Autodesk Fusion 360 part; units mm, degrees
(part 2 of 3)
  spline S192 degree 2 poles (79.2808, -26.577) (79.6552, -26.1242) (80.3974, -26.1242) knots 0 0 0 1 1 1
  spline S193 degree 2 poles (81.8524, -24.5056) (82.3952, -24.5056) (82.6732, -24.3274) knots 0 0 0 1 1 1
  spline S194 degree 2 poles (82.6732, -24.3274) (82.9511, -24.1492) (82.9511, -23.7471) knots 0 0 0 1 1 1
  spline S195 degree 2 poles (82.9511, -23.7471) (82.9511, -23.3481) (82.6748, -23.1732) knots 0 0 0 1 1 1
  spline S196 degree 2 poles (82.6748, -23.1732) (82.3985, -22.9983) (81.8524, -22.9983) knots 0 0 0 1 1 1
  spline S197 degree 2 poles (81.8524, -22.9983) (81.3097, -22.9983) (81.0383, -23.1748) knots 0 0 0 1 1 1
  spline S198 degree 2 poles (81.0383, -23.1748) (80.7669, -23.3514) (80.7669, -23.7536) knots 0 0 0 1 1 1
  spline S199 degree 2 poles (80.7669, -23.7536) (80.7669, -24.1525) (81.0366, -24.3291) knots 0 0 0 1 1 1
  spline S200 degree 2 poles (81.0366, -24.3291) (81.3064, -24.5056) (81.8524, -24.5056) knots 0 0 0 1 1 1
  spline S201 degree 2 poles (81.8524, -21.9781) (82.7451, -21.9781) (83.2486, -22.449) knots 0 0 0 1 1 1
  spline S202 degree 2 poles (83.2486, -22.449) (83.7522, -22.9198) (83.7522, -23.7601) knots 0 0 0 1 1 1
  spline S203 degree 2 poles (83.7522, -23.7601) (83.7522, -24.2866) (83.5217, -24.6887) knots 0 0 0 1 1 1
  spline S204 degree 2 poles (83.5217, -24.6887) (83.2911, -25.0909) (82.8595, -25.3067) knots 0 0 0 1 1 1
  spline S205 degree 2 poles (82.8595, -25.3067) (82.4279, -25.5225) (81.8524, -25.5225) knots 0 0 0 1 1 1
  spline S206 degree 2 poles (81.8524, -25.5225) (80.9565, -25.5225) (80.4595, -25.055) knots 0 0 0 1 1 1
  spline S207 degree 2 poles (80.4595, -25.055) (79.9625, -24.5874) (79.9625, -23.7405) knots 0 0 0 1 1 1
  spline S208 degree 2 poles (79.9625, -23.7405) (79.9625, -23.2141) (80.1914, -22.8119) knots 0 0 0 1 1 1
  spline S209 degree 2 poles (80.1914, -22.8119) (80.4203, -22.4097) (80.8486, -22.1939) knots 0 0 0 1 1 1
  spline S210 degree 2 poles (80.8486, -22.1939) (81.277, -21.9781) (81.8524, -21.9781) knots 0 0 0 1 1 1
  line L170 (83.6868, -18.1492) -> (82.4083, -18.4304)
  line L171 (82.4083, -18.4304) -> (80.793, -18.8097)
  line L172 (80.793, -18.8097) -> (80.793, -18.8326)
  line L173 (80.793, -18.8326) -> (83.6868, -19.4996)
  line L174 (83.6868, -19.4996) -> (83.6868, -20.5721)
  line L175 (83.6868, -20.5721) -> (80.0312, -21.6119)
  line L176 (80.0312, -21.6119) -> (80.0312, -20.6179)
  line L177 (80.0312, -20.6179) -> (81.6497, -20.1961)
  spline S211 degree 2 poles (81.6497, -20.1961) (82.0846, -20.0947) (82.8497, -19.9901) knots 0 0 0 1 1 1
  line L178 (82.8497, -19.9901) -> (82.8497, -19.9705)
  spline S212 degree 2 poles (82.8497, -19.9705) (82.6012, -19.9574) (82.0617, -19.856) knots 0 0 0 1 1 1
  line L179 (82.0617, -19.856) -> (81.7838, -19.8037)
  line L180 (81.7838, -19.8037) -> (80.0312, -19.3525)
  line L181 (80.0312, -19.3525) -> (80.0312, -18.2539)
  line L182 (80.0312, -18.2539) -> (81.7838, -17.8255)
  spline S213 degree 2 poles (81.7838, -17.8255) (81.8557, -17.8124) (81.9963, -17.7847) knots 0 0 0 1 1 1
  spline S214 degree 2 poles (81.9963, -17.7847) (82.1369, -17.7569) (82.2955, -17.7307) knots 0 0 0 1 1 1
  spline S215 degree 2 poles (82.2955, -17.7307) (82.4541, -17.7045) (82.6061, -17.6833) knots 0 0 0 1 1 1
  spline S216 degree 2 poles (82.6061, -17.6833) (82.7582, -17.662) (82.8497, -17.6588) knots 0 0 0 1 1 1
  line L183 (82.8497, -17.6588) -> (82.8497, -17.6392)
  spline S217 degree 2 poles (82.8497, -17.6392) (82.6143, -17.6097) (82.2039, -17.5345) knots 0 0 0 1 1 1
  spline S218 degree 2 poles (82.2039, -17.5345) (81.7936, -17.4593) (81.6497, -17.4266) knots 0 0 0 1 1 1
  line L184 (81.6497, -17.4266) -> (80.0312, -16.9885)
  line L185 (80.0312, -16.9885) -> (80.0312, -16.0108)
  line L186 (80.0312, -16.0108) -> (83.6868, -17.0637)
  line L187 (83.6868, -17.0637) -> (83.6868, -18.1492)
  spline S219 degree 2 poles (80.6721, -13.9084) (80.6721, -14.2255) (80.8732, -14.4054) knots 0 0 0 1 1 1
  spline S220 degree 2 poles (80.8732, -14.4054) (81.0742, -14.5852) (81.4437, -14.6114) knots 0 0 0 1 1 1
  line L188 (81.4437, -14.6114) -> (81.4437, -13.2119)
  spline S221 degree 2 poles (81.4437, -13.2119) (81.0742, -13.2184) (80.8732, -13.4048) knots 0 0 0 1 1 1
  spline S222 degree 2 poles (80.8732, -13.4048) (80.6721, -13.5912) (80.6721, -13.9084) knots 0 0 0 1 1 1
  spline S223 degree 2 poles (83.7522, -13.7678) (83.7522, -14.6506) (83.265, -15.1476) knots 0 0 0 1 1 1
  spline S224 degree 2 poles (83.265, -15.1476) (82.7778, -15.6446) (81.8851, -15.6446) knots 0 0 0 1 1 1
  spline S225 degree 2 poles (81.8851, -15.6446) (80.9663, -15.6446) (80.4644, -15.1852) knots 0 0 0 1 1 1
  spline S226 degree 2 poles (80.4644, -15.1852) (79.9625, -14.7258) (79.9625, -13.9149) knots 0 0 0 1 1 1
  spline S227 degree 2 poles (79.9625, -13.9149) (79.9625, -13.14) (80.4039, -12.7084) knots 0 0 0 1 1 1
  spline S228 degree 2 poles (80.4039, -12.7084) (80.8454, -12.2768) (81.6236, -12.2768) knots 0 0 0 1 1 1
  line L189 (81.6236, -12.2768) -> (82.1075, -12.2768)
  line L190 (82.1075, -12.2768) -> (82.1075, -14.6342)
  spline S229 degree 2 poles (82.1075, -14.6342) (82.5326, -14.6179) (82.7712, -14.3825) knots 0 0 0 1 1 1
  spline S230 degree 2 poles (82.7712, -14.3825) (83.0099, -14.1471) (83.0099, -13.722) knots 0 0 0 1 1 1
  spline S231 degree 2 poles (83.0099, -13.722) (83.0099, -13.3917) (82.9413, -13.0975) knots 0 0 0 1 1 1
  spline S232 degree 2 poles (82.9413, -13.0975) (82.8726, -12.8032) (82.7222, -12.4827) knots 0 0 0 1 1 1
  line L191 (82.7222, -12.4827) -> (83.4939, -12.4827)
  spline S233 degree 2 poles (83.4939, -12.4827) (83.6246, -12.7443) (83.6884, -13.0419) knots 0 0 0 1 1 1
  spline S234 degree 2 poles (83.6884, -13.0419) (83.7522, -13.3394) (83.7522, -13.7678) knots 0 0 0 1 1 1
  spline S235 degree 2 poles (79.9625, -9.4255) (79.9625, -9.2228) (79.992, -9.0887) knots 0 0 0 1 1 1
  line L192 (79.992, -9.0887) -> (80.9271, -9.1639)
  spline S236 degree 2 poles (80.9271, -9.1639) (80.8944, -9.2849) (80.8944, -9.4582) knots 0 0 0 1 1 1
  spline S237 degree 2 poles (80.8944, -9.4582) (80.8944, -9.9356) (81.1396, -10.2021) knots 0 0 0 1 1 1
  spline S238 degree 2 poles (81.1396, -10.2021) (81.3849, -10.4686) (81.8263, -10.4686) knots 0 0 0 1 1 1
  line L193 (81.8263, -10.4686) -> (83.6868, -10.4686)
  line L194 (83.6868, -10.4686) -> (83.6868, -11.4659)
  line L195 (83.6868, -11.4659) -> (80.0312, -11.4659)
  line L196 (80.0312, -11.4659) -> (80.0312, -10.7105)
  line L197 (80.0312, -10.7105) -> (80.6459, -10.5634)
  line L198 (80.6459, -10.5634) -> (80.6459, -10.5144)
  spline S239 degree 2 poles (80.6459, -10.5144) (80.3385, -10.3443) (80.1505, -10.055) knots 0 0 0 1 1 1
  spline S240 degree 2 poles (80.1505, -10.055) (79.9625, -9.7656) (79.9625, -9.4255) knots 0 0 0 1 1 1
  line L199 (86.415, -25.4932) -> (89.5081, -25.4932)
  spline S241 degree 2 poles (89.5081, -25.4932) (90.0378, -25.4932) (90.4368, -25.7303) knots 0 0 0 1 1 1
  spline S242 degree 2 poles (90.4368, -25.7303) (90.8357, -25.9673) (91.0482, -26.4153) knots 0 0 0 1 1 1
  spline S243 degree 2 poles (91.0482, -26.4153) (91.2607, -26.8632) (91.2607, -27.4747) knots 0 0 0 1 1 1
  spline S244 degree 2 poles (91.2607, -27.4747) (91.2607, -28.3968) (90.7883, -28.9068) knots 0 0 0 1 1 1
  spline S245 degree 2 poles (90.7883, -28.9068) (90.3158, -29.4169) (89.4951, -29.4169) knots 0 0 0 1 1 1
  line L200 (89.4951, -29.4169) -> (86.415, -29.4169)
  line L201 (86.415, -29.4169) -> (86.415, -28.4066)
  line L202 (86.415, -28.4066) -> (89.3414, -28.4066)
  spline S246 degree 2 poles (89.3414, -28.4066) (89.894, -28.4066) (90.1523, -28.1842) knots 0 0 0 1 1 1
  spline S247 degree 2 poles (90.1523, -28.1842) (90.4106, -27.9619) (90.4106, -27.4485) knots 0 0 0 1 1 1
  spline S248 degree 2 poles (90.4106, -27.4485) (90.4106, -26.9515) (90.1506, -26.7276) knots 0 0 0 1 1 1
  spline S249 degree 2 poles (90.1506, -26.7276) (89.8907, -26.5036) (89.3348, -26.5036) knots 0 0 0 1 1 1
  line L203 (89.3348, -26.5036) -> (86.415, -26.5036)
  line L204 (86.415, -26.5036) -> (86.415, -25.4932)
  spline S250 degree 2 poles (89.8678, -21.5009) (90.5152, -21.5009) (90.888, -21.9668) knots 0 0 0 1 1 1
  spline S251 degree 2 poles (90.888, -21.9668) (91.2607, -22.4327) (91.2607, -23.2632) knots 0 0 0 1 1 1
  spline S252 degree 2 poles (91.2607, -23.2632) (91.2607, -24.0284) (90.973, -24.6169) knots 0 0 0 1 1 1
  line L205 (90.973, -24.6169) -> (90.0313, -24.6169)
  spline S253 degree 2 poles (90.0313, -24.6169) (90.2471, -24.133) (90.3354, -23.7979) knots 0 0 0 1 1 1
  spline S254 degree 2 poles (90.3354, -23.7979) (90.4237, -23.4627) (90.4237, -23.1848) knots 0 0 0 1 1 1
  spline S255 degree 2 poles (90.4237, -23.1848) (90.4237, -22.8513) (90.2962, -22.6731) knots 0 0 0 1 1 1
  spline S256 degree 2 poles (90.2962, -22.6731) (90.1686, -22.4949) (89.9169, -22.4949) knots 0 0 0 1 1 1
  spline S257 degree 2 poles (89.9169, -22.4949) (89.7763, -22.4949) (89.6667, -22.5733) knots 0 0 0 1 1 1
  spline S258 degree 2 poles (89.6667, -22.5733) (89.5572, -22.6518) (89.4558, -22.8038) knots 0 0 0 1 1 1
  spline S259 degree 2 poles (89.4558, -22.8038) (89.3545, -22.9559) (89.1321, -23.4235) knots 0 0 0 1 1 1
  spline S260 degree 2 poles (89.1321, -23.4235) (88.9261, -23.8616) (88.7365, -24.0807) knots 0 0 0 1 1 1
  spline S261 degree 2 poles (88.7365, -24.0807) (88.5468, -24.2998) (88.2951, -24.4306) knots 0 0 0 1 1 1
  spline S262 degree 2 poles (88.2951, -24.4306) (88.0433, -24.5613) (87.7065, -24.5613) knots 0 0 0 1 1 1
  spline S263 degree 2 poles (87.7065, -24.5613) (87.0722, -24.5613) (86.7092, -24.1314) knots 0 0 0 1 1 1
  spline S264 degree 2 poles (86.7092, -24.1314) (86.3463, -23.7014) (86.3463, -22.9428) knots 0 0 0 1 1 1
  spline S265 degree 2 poles (86.3463, -22.9428) (86.3463, -22.5701) (86.4346, -22.2316) knots 0 0 0 1 1 1
  spline S266 degree 2 poles (86.4346, -22.2316) (86.5229, -21.8932) (86.6831, -21.5237) knots 0 0 0 1 1 1
  line L206 (86.6831, -21.5237) -> (87.4711, -21.8507)
  spline S267 degree 2 poles (87.4711, -21.8507) (87.3141, -22.2333) (87.252, -22.4834) knots 0 0 0 1 1 1
  spline S268 degree 2 poles (87.252, -22.4834) (87.1899, -22.7335) (87.1899, -22.9755) knots 0 0 0 1 1 1
  spline S269 degree 2 poles (87.1899, -22.9755) (87.1899, -23.2632) (87.3239, -23.4169) knots 0 0 0 1 1 1
  spline S270 degree 2 poles (87.3239, -23.4169) (87.458, -23.5706) (87.6738, -23.5706) knots 0 0 0 1 1 1
  spline S271 degree 2 poles (87.6738, -23.5706) (87.8079, -23.5706) (87.9076, -23.5085) knots 0 0 0 1 1 1
  spline S272 degree 2 poles (87.9076, -23.5085) (88.0073, -23.4464) (88.1005, -23.3107) knots 0 0 0 1 1 1
  spline S273 degree 2 poles (88.1005, -23.3107) (88.1937, -23.175) (88.4357, -22.6682) knots 0 0 0 1 1 1
  spline S274 degree 2 poles (88.4357, -22.6682) (88.7561, -21.9979) (89.0782, -21.7494) knots 0 0 0 1 1 1
  spline S275 degree 2 poles (89.0782, -21.7494) (89.4002, -21.5009) (89.8678, -21.5009) knots 0 0 0 1 1 1
  line L207 (86.415, -20.6344) -> (86.415, -19.1466)
  spline S276 degree 2 poles (86.415, -19.1466) (86.415, -18.1297) (86.7043, -17.6703) knots 0 0 0 1 1 1
  spline S277 degree 2 poles (86.7043, -17.6703) (86.9937, -17.2109) (87.6248, -17.2109) knots 0 0 0 1 1 1
  spline S278 degree 2 poles (87.6248, -17.2109) (88.0531, -17.2109) (88.3278, -17.412) knots 0 0 0 1 1 1
  spline S279 degree 2 poles (88.3278, -17.412) (88.6024, -17.6131) (88.658, -17.9466) knots 0 0 0 1 1 1
  line L208 (88.658, -17.9466) -> (88.6907, -17.9466)
  spline S280 degree 2 poles (88.6907, -17.9466) (88.7921, -17.4921) (89.07, -17.291) knots 0 0 0 1 1 1
  spline S281 degree 2 poles (89.07, -17.291) (89.3479, -17.09) (89.809, -17.09) knots 0 0 0 1 1 1
  spline S282 degree 2 poles (89.809, -17.09) (90.4629, -17.09) (90.8291, -17.5624) knots 0 0 0 1 1 1
  spline S283 degree 2 poles (90.8291, -17.5624) (91.1953, -18.0349) (91.1953, -18.8458) knots 0 0 0 1 1 1
  line L209 (91.1953, -18.8458) -> (91.1953, -20.6344)
  line L210 (91.1953, -20.6344) -> (86.415, -20.6344)
  line L211 (88.3081, -19.6207) -> (88.3081, -19.0322)
  spline S284 degree 2 poles (88.3081, -19.0322) (88.3081, -18.6202) (88.1806, -18.4355) knots 0 0 0 1 1 1
  spline S285 degree 2 poles (88.1806, -18.4355) (88.0531, -18.2507) (87.7588, -18.2507) knots 0 0 0 1 1 1
  spline S286 degree 2 poles (87.7588, -18.2507) (87.4842, -18.2507) (87.3648, -18.4518) knots 0 0 0 1 1 1
  spline S287 degree 2 poles (87.3648, -18.4518) (87.2455, -18.6529) (87.2455, -19.0878) knots 0 0 0 1 1 1
  line L212 (87.2455, -19.0878) -> (87.2455, -19.6207)
  line L213 (87.2455, -19.6207) -> (88.3081, -19.6207)
  line L214 (89.1125, -19.6207) -> (90.3583, -19.6207)
  line L215 (90.3583, -19.6207) -> (90.3583, -18.9603)
  spline S288 degree 2 poles (90.3583, -18.9603) (90.3583, -18.5417) (90.1981, -18.3423) knots 0 0 0 1 1 1
  spline S289 degree 2 poles (90.1981, -18.3423) (90.0378, -18.1428) (89.7076, -18.1428) knots 0 0 0 1 1 1
  spline S290 degree 2 poles (89.7076, -18.1428) (89.1125, -18.1428) (89.1125, -18.9929) knots 0 0 0 1 1 1
  line L216 (89.1125, -18.9929) -> (89.1125, -19.6207)
  spline S291 degree 2 poles (88.775, -9.3627) (89.9554, -9.3627) (90.5832, -10.0346) knots 0 0 0 1 1 1
  spline S292 degree 2 poles (90.5832, -10.0346) (91.211, -10.7066) (91.211, -11.9752) knots 0 0 0 1 1 1
  line L217 (91.211, -11.9752) -> (91.211, -13.3289)
  line L218 (91.211, -13.3289) -> (86.4306, -13.3289)
  line L219 (86.4306, -13.3289) -> (86.4306, -11.8281)
  spline S293 degree 2 poles (86.4306, -11.8281) (86.4306, -10.6575) (87.0486, -10.0101) knots 0 0 0 1 1 1
  spline S294 degree 2 poles (87.0486, -10.0101) (87.6666, -9.3627) (88.775, -9.3627) knots 0 0 0 1 1 1
  spline S295 degree 2 poles (88.8012, -10.4156) (87.2611, -10.4156) (87.2611, -11.7758) knots 0 0 0 1 1 1
  line L220 (87.2611, -11.7758) -> (87.2611, -12.3153)
  line L221 (87.2611, -12.3153) -> (90.3739, -12.3153)
  line L222 (90.3739, -12.3153) -> (90.3739, -11.8804)
  spline S296 degree 2 poles (90.3739, -11.8804) (90.3739, -10.4156) (88.8012, -10.4156) knots 0 0 0 1 1 1
  spline S297 degree 2 poles (87.2055, -6.3415) (87.2055, -6.9137) (87.6355, -7.2276) knots 0 0 0 1 1 1
  spline S298 degree 2 poles (87.6355, -7.2276) (88.0655, -7.5415) (88.8339, -7.5415) knots 0 0 0 1 1 1
  spline S299 degree 2 poles (88.8339, -7.5415) (90.4328, -7.5415) (90.4328, -6.3415) knots 0 0 0 1 1 1
  spline S300 degree 2 poles (90.4328, -6.3415) (90.4328, -5.8379) (90.181, -5.1218) knots 0 0 0 1 1 1
  line L223 (90.181, -5.1218) -> (91.0312, -5.1218)
  spline S301 degree 2 poles (91.0312, -5.1218) (91.2764, -5.7104) (91.2764, -6.4363) knots 0 0 0 1 1 1
  spline S302 degree 2 poles (91.2764, -6.4363) (91.2764, -7.4793) (90.6437, -8.0319) knots 0 0 0 1 1 1
  spline S303 degree 2 poles (90.6437, -8.0319) (90.011, -8.5845) (88.8273, -8.5845) knots 0 0 0 1 1 1
  spline S304 degree 2 poles (88.8273, -8.5845) (88.0818, -8.5845) (87.5211, -8.3131) knots 0 0 0 1 1 1
  spline S305 degree 2 poles (87.5211, -8.3131) (86.9603, -8.0417) (86.6611, -7.5333) knots 0 0 0 1 1 1
  spline S306 degree 2 poles (86.6611, -7.5333) (86.3619, -7.0248) (86.3619, -6.3415) knots 0 0 0 1 1 1
  spline S307 degree 2 poles (86.3619, -6.3415) (86.3619, -5.645) (86.6987, -4.942) knots 0 0 0 1 1 1
  line L224 (86.6987, -4.942) -> (87.5227, -5.269)
  spline S308 degree 2 poles (87.5227, -5.269) (87.3952, -5.5371) (87.3004, -5.8085) knots 0 0 0 1 1 1
  spline S309 degree 2 poles (87.3004, -5.8085) (87.2055, -6.0799) (87.2055, -6.3415) knots 0 0 0 1 1 1
  line L225 (91.0279, -57.901) -> (91.0279, -58.9146)
  line L226 (91.0279, -58.9146) -> (87.0912, -58.9146)
  line L227 (87.0912, -58.9146) -> (87.0912, -60.2127)
  line L228 (87.0912, -60.2127) -> (86.2476, -60.2127)
  line L229 (86.2476, -60.2127) -> (86.2476, -56.6029)
  line L230 (86.2476, -56.6029) -> (87.0912, -56.6029)
  line L231 (87.0912, -56.6029) -> (87.0912, -57.901)
  line L232 (87.0912, -57.901) -> (91.0279, -57.901)
  line L233 (91.0279, -54.0231) -> (91.0279, -55.0367)
  line L234 (91.0279, -55.0367) -> (87.0912, -55.0367)
  line L235 (87.0912, -55.0367) -> (87.0912, -56.3348)
  line L236 (87.0912, -56.3348) -> (86.2476, -56.3348)
  line L237 (86.2476, -56.3348) -> (86.2476, -52.725)
  line L238 (86.2476, -52.725) -> (87.0912, -52.725)
  line L239 (87.0912, -52.725) -> (87.0912, -54.0231)
  line L240 (87.0912, -54.0231) -> (91.0279, -54.0231)
  line L241 (91.0279, -51.9893) -> (86.2476, -51.9893)
  line L242 (86.2476, -51.9893) -> (86.2476, -50.9757)
  line L243 (86.2476, -50.9757) -> (90.1909, -50.9757)
  line L244 (90.1909, -50.9757) -> (90.1909, -49.0367)
  line L245 (90.1909, -49.0367) -> (91.0279, -49.0367)
  line L246 (91.0279, -49.0367) -> (91.0279, -51.9893)
  line L247 (88.4448, -91.7143) -> (88.4448, -91.3873)
  spline S310 degree 2 poles (88.4448, -91.3873) (88.4448, -90.9067) (88.2846, -90.6778) knots 0 0 0 1 1 1
  spline S311 degree 2 poles (88.2846, -90.6778) (88.1244, -90.4489) (87.781, -90.4489) knots 0 0 0 1 1 1
  spline S312 degree 2 poles (87.781, -90.4489) (87.441, -90.4489) (87.2971, -90.6827) knots 0 0 0 1 1 1
  spline S313 degree 2 poles (87.2971, -90.6827) (87.1532, -90.9165) (87.1532, -91.4069) knots 0 0 0 1 1 1
  line L248 (87.1532, -91.4069) -> (87.1532, -91.7143)
  line L249 (87.1532, -91.7143) -> (88.4448, -91.7143)
  line L250 (89.2688, -91.7143) -> (91.1031, -91.7143)
  line L251 (91.1031, -91.7143) -> (91.1031, -92.7279)
  line L252 (91.1031, -92.7279) -> (86.3227, -92.7279)
  line L253 (86.3227, -92.7279) -> (86.3227, -91.335)
  spline S314 degree 2 poles (86.3227, -91.335) (86.3227, -90.3606) (86.6775, -89.893) knots 0 0 0 1 1 1
  spline S315 degree 2 poles (86.6775, -89.893) (87.0323, -89.4255) (87.7549, -89.4255) knots 0 0 0 1 1 1
  spline S316 degree 2 poles (87.7549, -89.4255) (88.1767, -89.4255) (88.5053, -89.6576) knots 0 0 0 1 1 1
  spline S317 degree 2 poles (88.5053, -89.6576) (88.8339, -89.8898) (89.0203, -90.3148) knots 0 0 0 1 1 1
  spline S318 degree 2 poles (89.0203, -90.3148) (90.6323, -89.2358) (91.1031, -88.9088) knots 0 0 0 1 1 1
  line L254 (91.1031, -88.9088) -> (91.1031, -90.0336)
  line L255 (91.1031, -90.0336) -> (89.2688, -91.1748)
  line L256 (89.2688, -91.1748) -> (89.2688, -91.7143)
  spline S319 degree 2 poles (89.7756, -85.4854) (90.423, -85.4854) (90.7957, -85.9514) knots 0 0 0 1 1 1
  spline S320 degree 2 poles (90.7957, -85.9514) (91.1685, -86.4173) (91.1685, -87.2478) knots 0 0 0 1 1 1
  spline S321 degree 2 poles (91.1685, -87.2478) (91.1685, -88.0129) (90.8808, -88.6015) knots 0 0 0 1 1 1
  line L257 (90.8808, -88.6015) -> (89.9391, -88.6015)
  spline S322 degree 2 poles (89.9391, -88.6015) (90.1549, -88.1176) (90.2432, -87.7824) knots 0 0 0 1 1 1
  spline S323 degree 2 poles (90.2432, -87.7824) (90.3314, -87.4473) (90.3314, -87.1693) knots 0 0 0 1 1 1
  spline S324 degree 2 poles (90.3314, -87.1693) (90.3314, -86.8358) (90.2039, -86.6576) knots 0 0 0 1 1 1
  spline S325 degree 2 poles (90.2039, -86.6576) (90.0764, -86.4794) (89.8246, -86.4794) knots 0 0 0 1 1 1
  spline S326 degree 2 poles (89.8246, -86.4794) (89.684, -86.4794) (89.5745, -86.5579) knots 0 0 0 1 1 1
  spline S327 degree 2 poles (89.5745, -86.5579) (89.465, -86.6364) (89.3636, -86.7884) knots 0 0 0 1 1 1
  spline S328 degree 2 poles (89.3636, -86.7884) (89.2622, -86.9405) (89.0399, -87.408) knots 0 0 0 1 1 1
  spline S329 degree 2 poles (89.0399, -87.408) (88.8339, -87.8462) (88.6442, -88.0652) knots 0 0 0 1 1 1
  spline S330 degree 2 poles (88.6442, -88.0652) (88.4546, -88.2843) (88.2028, -88.4151) knots 0 0 0 1 1 1
  spline S331 degree 2 poles (88.2028, -88.4151) (87.9511, -88.5459) (87.6143, -88.5459) knots 0 0 0 1 1 1
  spline S332 degree 2 poles (87.6143, -88.5459) (86.9799, -88.5459) (86.617, -88.1159) knots 0 0 0 1 1 1
  spline S333 degree 2 poles (86.617, -88.1159) (86.2541, -87.686) (86.2541, -86.9274) knots 0 0 0 1 1 1
  spline S334 degree 2 poles (86.2541, -86.9274) (86.2541, -86.5546) (86.3423, -86.2162) knots 0 0 0 1 1 1
  spline S335 degree 2 poles (86.3423, -86.2162) (86.4306, -85.8778) (86.5908, -85.5083) knots 0 0 0 1 1 1
  line L258 (86.5908, -85.5083) -> (87.3788, -85.8353)
  spline S336 degree 2 poles (87.3788, -85.8353) (87.2219, -86.2178) (87.1598, -86.468) knots 0 0 0 1 1 1
  spline S337 degree 2 poles (87.1598, -86.468) (87.0976, -86.7181) (87.0976, -86.9601) knots 0 0 0 1 1 1
  spline S338 degree 2 poles (87.0976, -86.9601) (87.0976, -87.2478) (87.2317, -87.4015) knots 0 0 0 1 1 1
  spline S339 degree 2 poles (87.2317, -87.4015) (87.3658, -87.5552) (87.5816, -87.5552) knots 0 0 0 1 1 1
  spline S340 degree 2 poles (87.5816, -87.5552) (87.7156, -87.5552) (87.8154, -87.493) knots 0 0 0 1 1 1
  spline S341 degree 2 poles (87.8154, -87.493) (87.9151, -87.4309) (88.0083, -87.2952) knots 0 0 0 1 1 1
  spline S342 degree 2 poles (88.0083, -87.2952) (88.1015, -87.1595) (88.3434, -86.6527) knots 0 0 0 1 1 1
  spline S343 degree 2 poles (88.3434, -86.6527) (88.6639, -85.9824) (88.9859, -85.7339) knots 0 0 0 1 1 1
  spline S344 degree 2 poles (88.9859, -85.7339) (89.308, -85.4854) (89.7756, -85.4854) knots 0 0 0 1 1 1
  line L259 (91.1031, -81.6108) -> (91.1031, -84.9524)
  line L260 (91.1031, -84.9524) -> (90.4001, -84.9524)
  line L261 (90.4001, -84.9524) -> (89.187, -83.7524)
  spline S345 degree 2 poles (89.187, -83.7524) (88.641, -83.2195) (88.4301, -83.056) knots 0 0 0 1 1 1
  spline S346 degree 2 poles (88.4301, -83.056) (88.2192, -82.8925) (88.0393, -82.8206) knots 0 0 0 1 1 1
  spline S347 degree 2 poles (88.0393, -82.8206) (87.8595, -82.7486) (87.6666, -82.7486) knots 0 0 0 1 1 1
  spline S348 degree 2 poles (87.6666, -82.7486) (87.3788, -82.7486) (87.2382, -82.9072) knots 0 0 0 1 1 1
  spline S349 degree 2 poles (87.2382, -82.9072) (87.0976, -83.0658) (87.0976, -83.3306) knots 0 0 0 1 1 1
  spline S350 degree 2 poles (87.0976, -83.3306) (87.0976, -83.6086) (87.2252, -83.8702) knots 0 0 0 1 1 1
  spline S351 degree 2 poles (87.2252, -83.8702) (87.3527, -84.1317) (87.5881, -84.4162) knots 0 0 0 1 1 1
  line L262 (87.5881, -84.4162) -> (86.9374, -84.9655)
  spline S352 degree 2 poles (86.9374, -84.9655) (86.6366, -84.6124) (86.5124, -84.3802) knots 0 0 0 1 1 1
  spline S353 degree 2 poles (86.5124, -84.3802) (86.3881, -84.1481) (86.3211, -83.8734) knots 0 0 0 1 1 1
  spline S354 degree 2 poles (86.3211, -83.8734) (86.2541, -83.5988) (86.2541, -83.2587) knots 0 0 0 1 1 1
  spline S355 degree 2 poles (86.2541, -83.2587) (86.2541, -82.8108) (86.4175, -82.4674) knots 0 0 0 1 1 1
  spline S356 degree 2 poles (86.4175, -82.4674) (86.581, -82.1241) (86.8753, -81.9345) knots 0 0 0 1 1 1
  spline S357 degree 2 poles (86.8753, -81.9345) (87.1696, -81.7448) (87.5489, -81.7448) knots 0 0 0 1 1 1
  spline S358 degree 2 poles (87.5489, -81.7448) (87.8791, -81.7448) (88.1685, -81.8609) knots 0 0 0 1 1 1
  spline S359 degree 2 poles (88.1685, -81.8609) (88.4579, -81.977) (88.762, -82.2206) knots 0 0 0 1 1 1
  spline S360 degree 2 poles (88.762, -82.2206) (89.066, -82.4642) (89.6284, -83.0789) knots 0 0 0 1 1 1
  line L263 (89.6284, -83.0789) -> (90.2072, -83.6936)
  line L264 (90.2072, -83.6936) -> (90.253, -83.6936)
  line L265 (90.253, -83.6936) -> (90.253, -81.6108)
  line L266 (90.253, -81.6108) -> (91.1031, -81.6108)
  spline S361 degree 2 poles (87.3919, -77.9748) (87.8399, -77.9748) (88.1538, -78.2462) knots 0 0 0 1 1 1
  spline S362 degree 2 poles (88.1538, -78.2462) (88.4677, -78.5176) (88.5854, -79.008) knots 0 0 0 1 1 1
  line L267 (88.5854, -79.008) -> (88.605, -79.008)
  spline S363 degree 2 poles (88.605, -79.008) (88.6769, -78.4293) (88.9565, -78.1317) knots 0 0 0 1 1 1
  spline S364 degree 2 poles (88.9565, -78.1317) (89.2361, -77.8342) (89.7102, -77.8342) knots 0 0 0 1 1 1
  spline S365 degree 2 poles (89.7102, -77.8342) (90.4001, -77.8342) (90.7843, -78.3345) knots 0 0 0 1 1 1
  spline S366 degree 2 poles (90.7843, -78.3345) (91.1685, -78.8347) (91.1685, -79.7633) knots 0 0 0 1 1 1
  spline S367 degree 2 poles (91.1685, -79.7633) (91.1685, -80.5415) (90.9102, -81.1432) knots 0 0 0 1 1 1
  line L268 (90.9102, -81.1432) -> (90.0502, -81.1432)
  spline S368 degree 2 poles (90.0502, -81.1432) (90.1908, -80.8652) (90.2791, -80.5317) knots 0 0 0 1 1 1
  spline S369 degree 2 poles (90.2791, -80.5317) (90.3674, -80.1982) (90.3674, -79.8712) knots 0 0 0 1 1 1
  spline S370 degree 2 poles (90.3674, -79.8712) (90.3674, -79.371) (90.1974, -79.1323) knots 0 0 0 1 1 1
  spline S371 degree 2 poles (90.1974, -79.1323) (90.0273, -78.8936) (89.6513, -78.8936) knots 0 0 0 1 1 1
  spline S372 degree 2 poles (89.6513, -78.8936) (89.3145, -78.8936) (89.1739, -79.1682) knots 0 0 0 1 1 1
  spline S373 degree 2 poles (89.1739, -79.1682) (89.0333, -79.4429) (89.0333, -80.0445) knots 0 0 0 1 1 1
  line L269 (89.0333, -80.0445) -> (89.0333, -80.4075)
  line L270 (89.0333, -80.4075) -> (88.2584, -80.4075)
  line L271 (88.2584, -80.4075) -> (88.2584, -80.038)
  spline S374 degree 2 poles (88.2584, -80.038) (88.2584, -79.4821) (88.1129, -79.2255) knots 0 0 0 1 1 1
  spline S375 degree 2 poles (88.1129, -79.2255) (87.9674, -78.9688) (87.6143, -78.9688) knots 0 0 0 1 1 1
  spline S376 degree 2 poles (87.6143, -78.9688) (87.0715, -78.9688) (87.0715, -79.6489) knots 0 0 0 1 1 1
  spline S377 degree 2 poles (87.0715, -79.6489) (87.0715, -79.8843) (87.15, -80.1279) knots 0 0 0 1 1 1
  spline S378 degree 2 poles (87.15, -80.1279) (87.2284, -80.3715) (87.4214, -80.6691) knots 0 0 0 1 1 1
  line L272 (87.4214, -80.6691) -> (86.7249, -81.1366)
  spline S379 degree 2 poles (86.7249, -81.1366) (86.2541, -80.4827) (86.2541, -79.577) knots 0 0 0 1 1 1
  spline S380 degree 2 poles (86.2541, -79.577) (86.2541, -78.8347) (86.5549, -78.4048) knots 0 0 0 1 1 1
  spline S381 degree 2 poles (86.5549, -78.4048) (86.8557, -77.9748) (87.3919, -77.9748) knots 0 0 0 1 1 1
  line L273 (91.1031, -73.9661) -> (91.1031, -77.3078)
  line L274 (91.1031, -77.3078) -> (90.4001, -77.3078)
  line L275 (90.4001, -77.3078) -> (89.187, -76.1078)
  spline S382 degree 2 poles (89.187, -76.1078) (88.641, -75.5748) (88.4301, -75.4113) knots 0 0 0 1 1 1
  spline S383 degree 2 poles (88.4301, -75.4113) (88.2192, -75.2478) (88.0393, -75.1759) knots 0 0 0 1 1 1
  spline S384 degree 2 poles (88.0393, -75.1759) (87.8595, -75.1039) (87.6666, -75.1039) knots 0 0 0 1 1 1
  spline S385 degree 2 poles (87.6666, -75.1039) (87.3788, -75.1039) (87.2382, -75.2625) knots 0 0 0 1 1 1
  spline S386 degree 2 poles (87.2382, -75.2625) (87.0976, -75.4211) (87.0976, -75.686) knots 0 0 0 1 1 1
  spline S387 degree 2 poles (87.0976, -75.686) (87.0976, -75.9639) (87.2252, -76.2255) knots 0 0 0 1 1 1
  spline S388 degree 2 poles (87.2252, -76.2255) (87.3527, -76.487) (87.5881, -76.7715) knots 0 0 0 1 1 1
  line L276 (87.5881, -76.7715) -> (86.9374, -77.3208)
  spline S389 degree 2 poles (86.9374, -77.3208) (86.6366, -76.9677) (86.5124, -76.7355) knots 0 0 0 1 1 1
  spline S390 degree 2 poles (86.5124, -76.7355) (86.3881, -76.5034) (86.3211, -76.2287) knots 0 0 0 1 1 1
  spline S391 degree 2 poles (86.3211, -76.2287) (86.2541, -75.9541) (86.2541, -75.614) knots 0 0 0 1 1 1
  spline S392 degree 2 poles (86.2541, -75.614) (86.2541, -75.1661) (86.4175, -74.8227) knots 0 0 0 1 1 1
  spline S393 degree 2 poles (86.4175, -74.8227) (86.581, -74.4794) (86.8753, -74.2898) knots 0 0 0 1 1 1
  spline S394 degree 2 poles (86.8753, -74.2898) (87.1696, -74.1001) (87.5489, -74.1001) knots 0 0 0 1 1 1
  spline S395 degree 2 poles (87.5489, -74.1001) (87.8791, -74.1001) (88.1685, -74.2162) knots 0 0 0 1 1 1
  spline S396 degree 2 poles (88.1685, -74.2162) (88.4579, -74.3323) (88.762, -74.5759) knots 0 0 0 1 1 1
  spline S397 degree 2 poles (88.762, -74.5759) (89.066, -74.8195) (89.6284, -75.4342) knots 0 0 0 1 1 1
  line L277 (89.6284, -75.4342) -> (90.2072, -76.0489)
  line L278 (90.2072, -76.0489) -> (90.253, -76.0489)
  line L279 (90.253, -76.0489) -> (90.253, -73.9661)
  line L280 (90.253, -73.9661) -> (91.1031, -73.9661)
  spline S398 degree 2 poles (82.2535, -89.5798) (82.901, -89.5798) (83.2737, -90.0457) knots 0 0 0 1 1 1
  spline S399 degree 2 poles (83.2737, -90.0457) (83.6465, -90.5117) (83.6465, -91.3422) knots 0 0 0 1 1 1
  spline S400 degree 2 poles (83.6465, -91.3422) (83.6465, -92.1073) (83.3587, -92.6959) knots 0 0 0 1 1 1
  line L281 (83.3587, -92.6959) -> (82.417, -92.6959)
  spline S401 degree 2 poles (82.417, -92.6959) (82.6328, -92.2119) (82.7211, -91.8768) knots 0 0 0 1 1 1
  spline S402 degree 2 poles (82.7211, -91.8768) (82.8094, -91.5416) (82.8094, -91.2637) knots 0 0 0 1 1 1
  spline S403 degree 2 poles (82.8094, -91.2637) (82.8094, -90.9302) (82.6819, -90.752) knots 0 0 0 1 1 1
  spline S404 degree 2 poles (82.6819, -90.752) (82.5544, -90.5738) (82.3026, -90.5738) knots 0 0 0 1 1 1
  spline S405 degree 2 poles (82.3026, -90.5738) (82.162, -90.5738) (82.0525, -90.6523) knots 0 0 0 1 1 1
  spline S406 degree 2 poles (82.0525, -90.6523) (81.9429, -90.7307) (81.8416, -90.8828) knots 0 0 0 1 1 1
  spline S407 degree 2 poles (81.8416, -90.8828) (81.7402, -91.0348) (81.5178, -91.5024) knots 0 0 0 1 1 1
  spline S408 degree 2 poles (81.5178, -91.5024) (81.3119, -91.9406) (81.1222, -92.1596) knots 0 0 0 1 1 1
  spline S409 degree 2 poles (81.1222, -92.1596) (80.9326, -92.3787) (80.6808, -92.5095) knots 0 0 0 1 1 1
  spline S410 degree 2 poles (80.6808, -92.5095) (80.429, -92.6403) (80.0922, -92.6403) knots 0 0 0 1 1 1
  spline S411 degree 2 poles (80.0922, -92.6403) (79.4579, -92.6403) (79.095, -92.2103) knots 0 0 0 1 1 1
  spline S412 degree 2 poles (79.095, -92.2103) (78.732, -91.7803) (78.732, -91.0218) knots 0 0 0 1 1 1
  spline S413 degree 2 poles (78.732, -91.0218) (78.732, -90.649) (78.8203, -90.3106) knots 0 0 0 1 1 1
  spline S414 degree 2 poles (78.8203, -90.3106) (78.9086, -89.9722) (79.0688, -89.6027) knots 0 0 0 1 1 1
  line L282 (79.0688, -89.6027) -> (79.8568, -89.9297)
  spline S415 degree 2 poles (79.8568, -89.9297) (79.6999, -90.3122) (79.6377, -90.5624) knots 0 0 0 1 1 1
  spline S416 degree 2 poles (79.6377, -90.5624) (79.5756, -90.8125) (79.5756, -91.0545) knots 0 0 0 1 1 1
  spline S417 degree 2 poles (79.5756, -91.0545) (79.5756, -91.3422) (79.7097, -91.4959) knots 0 0 0 1 1 1
  spline S418 degree 2 poles (79.7097, -91.4959) (79.8437, -91.6496) (80.0595, -91.6496) knots 0 0 0 1 1 1
  spline S419 degree 2 poles (80.0595, -91.6496) (80.1936, -91.6496) (80.2933, -91.5874) knots 0 0 0 1 1 1
  spline S420 degree 2 poles (80.2933, -91.5874) (80.393, -91.5253) (80.4862, -91.3896) knots 0 0 0 1 1 1
  spline S421 degree 2 poles (80.4862, -91.3896) (80.5794, -91.2539) (80.8214, -90.7471) knots 0 0 0 1 1 1
  spline S422 degree 2 poles (80.8214, -90.7471) (81.1418, -90.0768) (81.4639, -89.8283) knots 0 0 0 1 1 1
  spline S423 degree 2 poles (81.4639, -89.8283) (81.786, -89.5798) (82.2535, -89.5798) knots 0 0 0 1 1 1
  spline S424 degree 2 poles (80.5663, -87.2779) (80.5663, -87.5951) (80.7674, -87.7749) knots 0 0 0 1 1 1
  spline S425 degree 2 poles (80.7674, -87.7749) (80.9685, -87.9547) (81.338, -87.9809) knots 0 0 0 1 1 1
  line L283 (81.338, -87.9809) -> (81.338, -86.5814)
  spline S426 degree 2 poles (81.338, -86.5814) (80.9685, -86.588) (80.7674, -86.7743) knots 0 0 0 1 1 1
  spline S427 degree 2 poles (80.7674, -86.7743) (80.5663, -86.9607) (80.5663, -87.2779) knots 0 0 0 1 1 1
  spline S428 degree 2 poles (83.6465, -87.1373) (83.6465, -88.0201) (83.1593, -88.5171) knots 0 0 0 1 1 1
  spline S429 degree 2 poles (83.1593, -88.5171) (82.6721, -89.0141) (81.7794, -89.0141) knots 0 0 0 1 1 1
  spline S430 degree 2 poles (81.7794, -89.0141) (80.8606, -89.0141) (80.3587, -88.5547) knots 0 0 0 1 1 1
  spline S431 degree 2 poles (80.3587, -88.5547) (79.8568, -88.0953) (79.8568, -87.2844) knots 0 0 0 1 1 1
  spline S432 degree 2 poles (79.8568, -87.2844) (79.8568, -86.5095) (80.2982, -86.0779) knots 0 0 0 1 1 1
  spline S433 degree 2 poles (80.2982, -86.0779) (80.7396, -85.6463) (81.5178, -85.6463) knots 0 0 0 1 1 1
  line L284 (81.5178, -85.6463) -> (82.0018, -85.6463)
  line L285 (82.0018, -85.6463) -> (82.0018, -88.0038)
  spline S434 degree 2 poles (82.0018, -88.0038) (82.4268, -87.9874) (82.6655, -87.752) knots 0 0 0 1 1 1
  spline S435 degree 2 poles (82.6655, -87.752) (82.9042, -87.5166) (82.9042, -87.0915) knots 0 0 0 1 1 1
  spline S436 degree 2 poles (82.9042, -87.0915) (82.9042, -86.7613) (82.8356, -86.467) knots 0 0 0 1 1 1
  spline S437 degree 2 poles (82.8356, -86.467) (82.7669, -86.1727) (82.6165, -85.8523) knots 0 0 0 1 1 1
  line L286 (82.6165, -85.8523) -> (83.3881, -85.8523)
  spline S438 degree 2 poles (83.3881, -85.8523) (83.5189, -86.1139) (83.5827, -86.4114) knots 0 0 0 1 1 1
  spline S439 degree 2 poles (83.5827, -86.4114) (83.6465, -86.709) (83.6465, -87.1373) knots 0 0 0 1 1 1
  spline S440 degree 2 poles (79.8568, -82.7951) (79.8568, -82.5923) (79.8862, -82.4583) knots 0 0 0 1 1 1
  line L287 (79.8862, -82.4583) -> (80.8214, -82.5335)
  spline S441 degree 2 poles (80.8214, -82.5335) (80.7887, -82.6545) (80.7887, -82.8278) knots 0 0 0 1 1 1
  spline S442 degree 2 poles (80.7887, -82.8278) (80.7887, -83.3051) (81.0339, -83.5716) knots 0 0 0 1 1 1
  spline S443 degree 2 poles (81.0339, -83.5716) (81.2792, -83.8381) (81.7206, -83.8381) knots 0 0 0 1 1 1
  line L288 (81.7206, -83.8381) -> (83.5811, -83.8381)
  line L289 (83.5811, -83.8381) -> (83.5811, -84.8354)
  line L290 (83.5811, -84.8354) -> (79.9255, -84.8354)
  line L291 (79.9255, -84.8354) -> (79.9255, -84.0801)
  line L292 (79.9255, -84.0801) -> (80.5402, -83.9329)
  line L293 (80.5402, -83.9329) -> (80.5402, -83.8839)
  spline S444 degree 2 poles (80.5402, -83.8839) (80.2328, -83.7139) (80.0448, -83.4245) knots 0 0 0 1 1 1
  spline S445 degree 2 poles (80.0448, -83.4245) (79.8568, -83.1351) (79.8568, -82.7951) knots 0 0 0 1 1 1
  spline S446 degree 2 poles (78.9805, -81.837) (78.4933, -81.837) (78.4933, -81.2942) knots 0 0 0 1 1 1
  spline S447 degree 2 poles (78.4933, -81.2942) (78.4933, -80.7515) (78.9805, -80.7515) knots 0 0 0 1 1 1
  spline S448 degree 2 poles (78.9805, -80.7515) (79.2127, -80.7515) (79.3418, -80.8872) knots 0 0 0 1 1 1
  spline S449 degree 2 poles (79.3418, -80.8872) (79.471, -81.0228) (79.471, -81.2942) knots 0 0 0 1 1 1
  spline S450 degree 2 poles (79.471, -81.2942) (79.471, -81.837) (78.9805, -81.837) knots 0 0 0 1 1 1
  line L294 (83.5811, -80.7972) -> (83.5811, -81.7945)
  line L295 (83.5811, -81.7945) -> (79.9255, -81.7945)
  line L296 (79.9255, -81.7945) -> (79.9255, -80.7972)
  line L297 (79.9255, -80.7972) -> (83.5811, -80.7972)
  line L298 (83.5811, -77.4294) -> (83.0841, -77.6223)
  line L299 (83.0841, -77.6223) -> (83.0841, -77.6485)
  spline S451 degree 2 poles (83.0841, -77.6485) (83.4012, -77.9002) (83.5238, -78.1667) knots 0 0 0 1 1 1
  spline S452 degree 2 poles (83.5238, -78.1667) (83.6465, -78.4332) (83.6465, -78.8615) knots 0 0 0 1 1 1
  spline S453 degree 2 poles (83.6465, -78.8615) (83.6465, -79.388) (83.3456, -79.6904) knots 0 0 0 1 1 1
  spline S454 degree 2 poles (83.3456, -79.6904) (83.0448, -79.9929) (82.489, -79.9929) knots 0 0 0 1 1 1
  spline S455 degree 2 poles (82.489, -79.9929) (81.9069, -79.9929) (81.6307, -79.5858) knots 0 0 0 1 1 1
  spline S456 degree 2 poles (81.6307, -79.5858) (81.3544, -79.1787) (81.3249, -78.358) knots 0 0 0 1 1 1
  line L300 (81.3249, -78.358) -> (81.3053, -77.7237)
  line L301 (81.3053, -77.7237) -> (81.1451, -77.7237)
  spline S457 degree 2 poles (81.1451, -77.7237) (80.5892, -77.7237) (80.5892, -78.2926) knots 0 0 0 1 1 1
  spline S458 degree 2 poles (80.5892, -78.2926) (80.5892, -78.7308) (80.8541, -79.3226) knots 0 0 0 1 1 1
  line L302 (80.8541, -79.3226) -> (80.1805, -79.6528)
  spline S459 degree 2 poles (80.1805, -79.6528) (79.8503, -79.0218) (79.8503, -78.2534) knots 0 0 0 1 1 1
  spline S460 degree 2 poles (79.8503, -78.2534) (79.8503, -77.5177) (80.1707, -77.1253) knots 0 0 0 1 1 1
  spline S461 degree 2 poles (80.1707, -77.1253) (80.4911, -76.7329) (81.1451, -76.7329) knots 0 0 0 1 1 1
  line L303 (81.1451, -76.7329) -> (83.5811, -76.7329)
  line L304 (83.5811, -76.7329) -> (83.5811, -77.4294)
  line L305 (81.8873, -77.7237) -> (81.9004, -78.1095)
  spline S462 degree 2 poles (81.9004, -78.1095) (81.9135, -78.5444) (82.0574, -78.7569) knots 0 0 0 1 1 1
  spline S463 degree 2 poles (82.0574, -78.7569) (82.2012, -78.9694) (82.4955, -78.9694) knots 0 0 0 1 1 1
  spline S464 degree 2 poles (82.4955, -78.9694) (82.9173, -78.9694) (82.9173, -78.4855) knots 0 0 0 1 1 1
  spline S465 degree 2 poles (82.9173, -78.4855) (82.9173, -78.1389) (82.7178, -77.9313) knots 0 0 0 1 1 1
  spline S466 degree 2 poles (82.7178, -77.9313) (82.5184, -77.7237) (82.1881, -77.7237) knots 0 0 0 1 1 1
  line L306 (82.1881, -77.7237) -> (81.8873, -77.7237)
  line L307 (83.5811, -74.709) -> (83.5811, -75.7062)
  line L308 (83.5811, -75.7062) -> (78.4933, -75.7062)
  line L309 (78.4933, -75.7062) -> (78.4933, -74.709)
  line L310 (78.4933, -74.709) -> (83.5811, -74.709)
  line L311 (84.5897, -92.756) -> (85.1897, -92.756)
  line L312 (85.1897, -92.756) -> (85.1897, -37.8101)
  line L313 (85.1897, -37.8101) -> (84.5897, -37.8101)
  line L314 (84.5897, -37.8101) -> (84.5897, -92.756)
  line L315 (42.868, -78.8478) -> (42.868, -76.9715)
  line L316 (42.868, -76.9715) -> (51.632, -79.9508)
  line L317 (51.632, -79.9508) -> (51.632, -81.977)
  line L318 (51.632, -81.977) -> (42.868, -84.9503)
  line L319 (42.868, -84.9503) -> (42.868, -83.074)
  line L320 (42.868, -83.074) -> (48.0832, -81.4255)
  spline S467 degree 2 poles (48.0832, -81.4255) (48.5448, -81.2876) (49.1593, -81.1407) knots 0 0 0 1 1 1
  spline S468 degree 2 poles (49.1593, -81.1407) (49.7737, -80.9939) (50.0135, -80.9579) knots 0 0 0 1 1 1
  spline S469 degree 2 poles (50.0135, -80.9579) (49.462, -80.892) (48.0832, -80.5083) knots 0 0 0 1 1 1
  line L321 (48.0832, -80.5083) -> (42.868, -78.8478)
  spline S470 degree 2 poles (46.105, -73.2369) (46.105, -73.8184) (46.4737, -74.1481) knots 0 0 0 1 1 1
  spline S471 degree 2 poles (46.4737, -74.1481) (46.8424, -74.4778) (47.5198, -74.5257) knots 0 0 0 1 1 1
  line L322 (47.5198, -74.5257) -> (47.5198, -71.9601)
  spline S472 degree 2 poles (47.5198, -71.9601) (46.8424, -71.9721) (46.4737, -72.3138) knots 0 0 0 1 1 1
  spline S473 degree 2 poles (46.4737, -72.3138) (46.105, -72.6554) (46.105, -73.2369) knots 0 0 0 1 1 1
  spline S474 degree 2 poles (51.7519, -72.9792) (51.7519, -74.5977) (50.8587, -75.5089) knots 0 0 0 1 1 1
  spline S475 degree 2 poles (50.8587, -75.5089) (49.9655, -76.42) (48.329, -76.42) knots 0 0 0 1 1 1
  spline S476 degree 2 poles (48.329, -76.42) (46.6445, -76.42) (45.7244, -75.5778) knots 0 0 0 1 1 1
  spline S477 degree 2 poles (45.7244, -75.5778) (44.8042, -74.7356) (44.8042, -73.2489) knots 0 0 0 1 1 1
  spline S478 degree 2 poles (44.8042, -73.2489) (44.8042, -71.8282) (45.6135, -71.0369) knots 0 0 0 1 1 1
  spline S479 degree 2 poles (45.6135, -71.0369) (46.4228, -70.2456) (47.8495, -70.2456) knots 0 0 0 1 1 1
  line L323 (47.8495, -70.2456) -> (48.7366, -70.2456)
  line L324 (48.7366, -70.2456) -> (48.7366, -74.5677)
  spline S480 degree 2 poles (48.7366, -74.5677) (49.5159, -74.5377) (49.9535, -74.1061) knots 0 0 0 1 1 1
  spline S481 degree 2 poles (49.9535, -74.1061) (50.3911, -73.6745) (50.3911, -72.8952) knots 0 0 0 1 1 1
  spline S482 degree 2 poles (50.3911, -72.8952) (50.3911, -72.2898) (50.2653, -71.7503) knots 0 0 0 1 1 1
  spline S483 degree 2 poles (50.2653, -71.7503) (50.1394, -71.2108) (49.8636, -70.6233) knots 0 0 0 1 1 1
  line L325 (49.8636, -70.6233) -> (51.2783, -70.6233)
  spline S484 degree 2 poles (51.2783, -70.6233) (51.5181, -71.1029) (51.635, -71.6484) knots 0 0 0 1 1 1
  spline S485 degree 2 poles (51.635, -71.6484) (51.7519, -72.1939) (51.7519, -72.9792) knots 0 0 0 1 1 1
  spline S486 degree 2 poles (44.8042, -65.0184) (44.8042, -64.6467) (44.8582, -64.401) knots 0 0 0 1 1 1
  line L326 (44.8582, -64.401) -> (46.5726, -64.5388)
  spline S487 degree 2 poles (46.5726, -64.5388) (46.5127, -64.7606) (46.5127, -65.0783) knots 0 0 0 1 1 1
  spline S488 degree 2 poles (46.5127, -65.0783) (46.5127, -65.9535) (46.9623, -66.4421) knots 0 0 0 1 1 1
  spline S489 degree 2 poles (46.9623, -66.4421) (47.4119, -66.9307) (48.2211, -66.9307) knots 0 0 0 1 1 1
  line L327 (48.2211, -66.9307) -> (51.632, -66.9307)
  line L328 (51.632, -66.9307) -> (51.632, -68.759)
  line L329 (51.632, -68.759) -> (44.9301, -68.759)
  line L330 (44.9301, -68.759) -> (44.9301, -67.3742)
  line L331 (44.9301, -67.3742) -> (46.0571, -67.1045)
  line L332 (46.0571, -67.1045) -> (46.0571, -67.0146)
  spline S490 degree 2 poles (46.0571, -67.0146) (45.4936, -66.7029) (45.1489, -66.1723) knots 0 0 0 1 1 1
  spline S491 degree 2 poles (45.1489, -66.1723) (44.8042, -65.6418) (44.8042, -65.0184) knots 0 0 0 1 1 1
  spline S492 degree 2 poles (49.6418, -58.5083) (50.6729, -58.5083) (51.2124, -59.2247) knots 0 0 0 1 1 1
  spline S493 degree 2 poles (51.2124, -59.2247) (51.7519, -59.941) (51.7519, -61.3677) knots 0 0 0 1 1 1
  spline S494 degree 2 poles (51.7519, -61.3677) (51.7519, -62.099) (51.653, -62.6146) knots 0 0 0 1 1 1
  spline S495 degree 2 poles (51.653, -62.6146) (51.5541, -63.1301) (51.3623, -63.5797) knots 0 0 0 1 1 1
  line L333 (51.3623, -63.5797) -> (49.8516, -63.5797)
  spline S496 degree 2 poles (49.8516, -63.5797) (50.0914, -63.0702) (50.2533, -62.4317) knots 0 0 0 1 1 1
  spline S497 degree 2 poles (50.2533, -62.4317) (50.4151, -61.7933) (50.4151, -61.3078) knots 0 0 0 1 1 1
  spline S498 degree 2 poles (50.4151, -61.3078) (50.4151, -60.3127) (49.8396, -60.3127) knots 0 0 0 1 1 1
  spline S499 degree 2 poles (49.8396, -60.3127) (49.6238, -60.3127) (49.489, -60.4445) knots 0 0 0 1 1 1
  spline S500 degree 2 poles (49.489, -60.4445) (49.3541, -60.5764) (49.1832, -60.9001) knots 0 0 0 1 1 1
  spline S501 degree 2 poles (49.1832, -60.9001) (49.0124, -61.2238) (48.7846, -61.7633) knots 0 0 0 1 1 1
  spline S502 degree 2 poles (48.7846, -61.7633) (48.4609, -62.5366) (48.1851, -62.8993) knots 0 0 0 1 1 1
  spline S503 degree 2 poles (48.1851, -62.8993) (47.9094, -63.262) (47.5527, -63.4268) knots 0 0 0 1 1 1
  spline S504 degree 2 poles (47.5527, -63.4268) (47.196, -63.5917) (46.6745, -63.5917) knots 0 0 0 1 1 1
  spline S505 degree 2 poles (46.6745, -63.5917) (45.7813, -63.5917) (45.2928, -62.8993) knots 0 0 0 1 1 1
  spline S506 degree 2 poles (45.2928, -62.8993) (44.8042, -62.2069) (44.8042, -60.9361) knots 0 0 0 1 1 1
  spline S507 degree 2 poles (44.8042, -60.9361) (44.8042, -59.7252) (45.3317, -58.5802) knots 0 0 0 1 1 1
  line L334 (45.3317, -58.5802) -> (46.6505, -59.1317)
  spline S508 degree 2 poles (46.6505, -59.1317) (46.4347, -59.6353) (46.2969, -60.0729) knots 0 0 0 1 1 1
  spline S509 degree 2 poles (46.2969, -60.0729) (46.159, -60.5105) (46.159, -60.9661) knots 0 0 0 1 1 1
  spline S510 degree 2 poles (46.159, -60.9661) (46.159, -61.7753) (46.5966, -61.7753) knots 0 0 0 1 1 1
  spline S511 degree 2 poles (46.5966, -61.7753) (46.8424, -61.7753) (47.0222, -61.5146) knots 0 0 0 1 1 1
  spline S512 degree 2 poles (47.0222, -61.5146) (47.202, -61.2538) (47.5557, -60.3726) knots 0 0 0 1 1 1
  spline S513 degree 2 poles (47.5557, -60.3726) (47.8734, -59.5873) (48.1492, -59.2217) knots 0 0 0 1 1 1
  spline S514 degree 2 poles (48.1492, -59.2217) (48.4249, -58.856) (48.7846, -58.6822) knots 0 0 0 1 1 1
  spline S515 degree 2 poles (48.7846, -58.6822) (49.1443, -58.5083) (49.6418, -58.5083) knots 0 0 0 1 1 1
  line L335 (51.632, -52.8255) -> (50.7208, -53.1792)
  line L336 (50.7208, -53.1792) -> (50.7208, -53.2271)
  spline S516 degree 2 poles (50.7208, -53.2271) (51.3023, -53.6887) (51.5271, -54.1772) knots 0 0 0 1 1 1
  spline S517 degree 2 poles (51.5271, -54.1772) (51.7519, -54.6658) (51.7519, -55.4511) knots 0 0 0 1 1 1
  spline S518 degree 2 poles (51.7519, -55.4511) (51.7519, -56.4162) (51.2004, -56.9707) knots 0 0 0 1 1 1
  spline S519 degree 2 poles (51.2004, -56.9707) (50.6489, -57.5252) (49.6298, -57.5252) knots 0 0 0 1 1 1
  spline S520 degree 2 poles (49.6298, -57.5252) (48.5628, -57.5252) (48.0563, -56.7789) knots 0 0 0 1 1 1
  spline S521 degree 2 poles (48.0563, -56.7789) (47.5497, -56.0326) (47.4958, -54.5279) knots 0 0 0 1 1 1
  line L337 (47.4958, -54.5279) -> (47.4598, -53.365)
  line L338 (47.4598, -53.365) -> (47.1661, -53.365)
  spline S522 degree 2 poles (47.1661, -53.365) (46.147, -53.365) (46.147, -54.408) knots 0 0 0 1 1 1
  spline S523 degree 2 poles (46.147, -54.408) (46.147, -55.2113) (46.6326, -56.2963) knots 0 0 0 1 1 1
  line L339 (46.6326, -56.2963) -> (45.3977, -56.9018)
  spline S524 degree 2 poles (45.3977, -56.9018) (44.7922, -55.7448) (44.7922, -54.3361) knots 0 0 0 1 1 1
  spline S525 degree 2 poles (44.7922, -54.3361) (44.7922, -52.9873) (45.3797, -52.268) knots 0 0 0 1 1 1
  spline S526 degree 2 poles (45.3797, -52.268) (45.9672, -51.5486) (47.1661, -51.5486) knots 0 0 0 1 1 1
  line L340 (47.1661, -51.5486) -> (51.632, -51.5486)
  line L341 (51.632, -51.5486) -> (51.632, -52.8255)
  line L342 (48.5268, -53.365) -> (48.5508, -54.0723)
  spline S527 degree 2 poles (48.5508, -54.0723) (48.5748, -54.8696) (48.8386, -55.2593) knots 0 0 0 1 1 1
  spline S528 degree 2 poles (48.8386, -55.2593) (49.1023, -55.6489) (49.6418, -55.6489) knots 0 0 0 1 1 1
  spline S529 degree 2 poles (49.6418, -55.6489) (50.4151, -55.6489) (50.4151, -54.7617) knots 0 0 0 1 1 1
  spline S530 degree 2 poles (50.4151, -54.7617) (50.4151, -54.1263) (50.0495, -53.7456) knots 0 0 0 1 1 1
  spline S531 degree 2 poles (50.0495, -53.7456) (49.6838, -53.365) (49.0783, -53.365) knots 0 0 0 1 1 1
  line L343 (49.0783, -53.365) -> (48.5268, -53.365)
  line L344 (51.632, -46.1416) -> (51.632, -47.9999)
  line L345 (51.632, -47.9999) -> (44.4146, -47.9999)
  line L346 (44.4146, -47.9999) -> (44.4146, -50.3797)
  line L347 (44.4146, -50.3797) -> (42.868, -50.3797)
  line L348 (42.868, -50.3797) -> (42.868, -43.7617)
  line L349 (42.868, -43.7617) -> (44.4146, -43.7617)
  line L350 (44.4146, -43.7617) -> (44.4146, -46.1416)
  line L351 (44.4146, -46.1416) -> (51.632, -46.1416)
  spline S532 degree 2 poles (46.105, -39.7813) (46.105, -40.3628) (46.4737, -40.6925) knots 0 0 0 1 1 1
  spline S533 degree 2 poles (46.4737, -40.6925) (46.8424, -41.0222) (47.5198, -41.0702) knots 0 0 0 1 1 1
  line L352 (47.5198, -41.0702) -> (47.5198, -38.5045)
  spline S534 degree 2 poles (47.5198, -38.5045) (46.8424, -38.5165) (46.4737, -38.8582) knots 0 0 0 1 1 1
  spline S535 degree 2 poles (46.4737, -38.8582) (46.105, -39.1999) (46.105, -39.7813) knots 0 0 0 1 1 1
  spline S536 degree 2 poles (51.7519, -39.5236) (51.7519, -41.1421) (50.8587, -42.0533) knots 0 0 0 1 1 1
  spline S537 degree 2 poles (50.8587, -42.0533) (49.9655, -42.9644) (48.329, -42.9644) knots 0 0 0 1 1 1
  spline S538 degree 2 poles (48.329, -42.9644) (46.6445, -42.9644) (45.7244, -42.1222) knots 0 0 0 1 1 1
  spline S539 degree 2 poles (45.7244, -42.1222) (44.8042, -41.28) (44.8042, -39.7933) knots 0 0 0 1 1 1
  spline S540 degree 2 poles (44.8042, -39.7933) (44.8042, -38.3726) (45.6135, -37.5813) knots 0 0 0 1 1 1
  spline S541 degree 2 poles (45.6135, -37.5813) (46.4228, -36.7901) (47.8495, -36.7901) knots 0 0 0 1 1 1
  line L353 (47.8495, -36.7901) -> (48.7366, -36.7901)
  line L354 (48.7366, -36.7901) -> (48.7366, -41.1121)
  spline S542 degree 2 poles (48.7366, -41.1121) (49.5159, -41.0821) (49.9535, -40.6505) knots 0 0 0 1 1 1
  spline S543 degree 2 poles (49.9535, -40.6505) (50.3911, -40.2189) (50.3911, -39.4396) knots 0 0 0 1 1 1
  spline S544 degree 2 poles (50.3911, -39.4396) (50.3911, -38.8342) (50.2653, -38.2947) knots 0 0 0 1 1 1
  spline S545 degree 2 poles (50.2653, -38.2947) (50.1394, -37.7552) (49.8636, -37.1677) knots 0 0 0 1 1 1
  line L355 (49.8636, -37.1677) -> (51.2783, -37.1677)
  spline S546 degree 2 poles (51.2783, -37.1677) (51.5181, -37.6473) (51.635, -38.1928) knots 0 0 0 1 1 1
  spline S547 degree 2 poles (51.635, -38.1928) (51.7519, -38.7383) (51.7519, -39.5236) knots 0 0 0 1 1 1
  spline S548 degree 2 poles (44.8042, -31.5628) (44.8042, -31.1911) (44.8582, -30.9454) knots 0 0 0 1 1 1
  line L356 (44.8582, -30.9454) -> (46.5726, -31.0832)
  spline S549 degree 2 poles (46.5726, -31.0832) (46.5127, -31.305) (46.5127, -31.6227) knots 0 0 0 1 1 1
  spline S550 degree 2 poles (46.5127, -31.6227) (46.5127, -32.498) (46.9623, -32.9865) knots 0 0 0 1 1 1
  spline S551 degree 2 poles (46.9623, -32.9865) (47.4119, -33.4751) (48.2211, -33.4751) knots 0 0 0 1 1 1
  line L357 (48.2211, -33.4751) -> (51.632, -33.4751)
  line L358 (51.632, -33.4751) -> (51.632, -35.3034)
  line L359 (51.632, -35.3034) -> (44.9301, -35.3034)
  line L360 (44.9301, -35.3034) -> (44.9301, -33.9187)
  line L361 (44.9301, -33.9187) -> (46.0571, -33.6489)
  line L362 (46.0571, -33.6489) -> (46.0571, -33.559)
  spline S552 degree 2 poles (46.0571, -33.559) (45.4936, -33.2473) (45.1489, -32.7168) knots 0 0 0 1 1 1
  spline S553 degree 2 poles (45.1489, -32.7168) (44.8042, -32.1862) (44.8042, -31.5628) knots 0 0 0 1 1 1
  line L363 (51.632, -23.7279) -> (51.632, -25.5563)
  line L364 (51.632, -25.5563) -> (47.7176, -25.5563)
  spline S554 degree 2 poles (47.7176, -25.5563) (46.9922, -25.5563) (46.6296, -25.799) knots 0 0 0 1 1 1
  spline S555 degree 2 poles (46.6296, -25.799) (46.2669, -26.0418) (46.2669, -26.5633) knots 0 0 0 1 1 1
  spline S556 degree 2 poles (46.2669, -26.5633) (46.2669, -27.2647) (46.7824, -27.5824) knots 0 0 0 1 1 1
  spline S557 degree 2 poles (46.7824, -27.5824) (47.298, -27.9001) (48.4789, -27.9001) knots 0 0 0 1 1 1
  line L365 (48.4789, -27.9001) -> (51.632, -27.9001)
  line L366 (51.632, -27.9001) -> (51.632, -29.7285)
  line L367 (51.632, -29.7285) -> (44.9301, -29.7285)
  line L368 (44.9301, -29.7285) -> (44.9301, -28.3317)
  line L369 (44.9301, -28.3317) -> (45.7873, -28.086)
  line L370 (45.7873, -28.086) -> (45.7873, -27.9841)